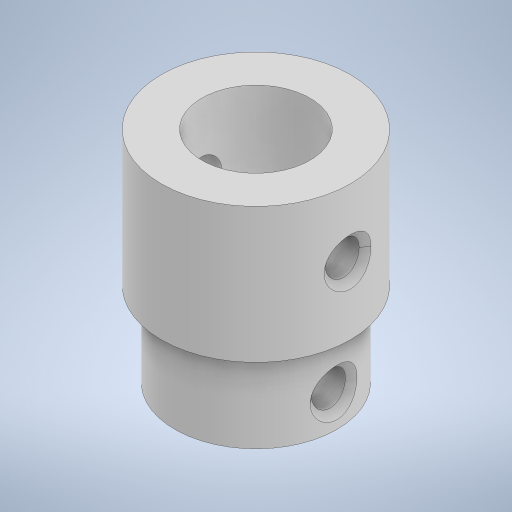
# Autodesk Inventor part: Acople2
Saved by Autodesk Inventor 2023 (Build 270158000, 158)
## iProperties
Created: 2022-12-24
Part Number: Acople2
Material: Genérico
Document SubType Name: Modeling
Designer: sergi
Density: 1 g/cm^3
Appearance: Valor por defecto
Author: sergi
Autodesk Inventor part; units mm, degrees
ref_plane "YZ Plane" through (0, 0, 0) normal (1, 0, 0) x (0, 1, 0)
ref_plane "XZ Plane" through (0, 0, 0) normal (0, 1, 0) x (-1, 0, 0)
ref_plane "XY Plane" through (0, 0, 0) normal (0, 0, 1) x (1, 0, 0)
sketch "Boceto1" plane through (0, 0, 0) normal (0, 1, 0) x (-1, 0, 0)
  circle A0 centre (0, 0) radius 7
  circle A1 centre (0, 0) radius 4
  dimension "d0" = 14
  dimension "d1" = 8
  constraints: 2 centre point, 2 coincident
  measures "d0" diameter of A0
  measures "d1" diameter of A1
extrude "Extrusión1" add sketch "Boceto1" along normal blind 10 contours A0 | A1
sketch "Boceto4" plane through (0, 10, 0) normal (0, 1, 0) x (1, 0, 0)
  circle A0 centre (0, 0) radius 4
  line L0 (0, 4) -> (0, -4)
  line L1 (-1.5, 4) -> (-1.5, -4)
  point P0 (-1.5, 3.7081)
  point P1 (-1.5, -3.7081)
  dimension "d21" = 8
  dimension "d45" = 1.5
  constraints: 4 end point, 2 point on circle, 1 centre point, 1 coincident, 1 parallel, 1 vertical
  measures "d21" diameter of A0
  measures "d45" distance between parallel lines of L0 L1
extrude "Extrusión2" cut sketch "Boceto4" against normal blind 8
sketch "Boceto5" plane through (0, 0, 0) normal (0, -1, 0) x (1, 0, 0)
  circle A0 centre (0, 0) radius 6
  dimension "d24" = 12
  constraints: 1 centre point, 1 coincident
  measures "d24" diameter of A0
extrude "Extrusión3" add sketch "Boceto5" along normal blind 6.25
sketch "Boceto11" plane through (0, 0, 0) normal (1, 0, 0) x (0, 1, 0)
  line L0 (-1.5, 0) -> (-1.5, 2.5882)
  line L1 (-1.5, 0) -> (-1.5, 2.5882)
  line L2 (0, 0) -> (-1.5, 0)
  line L3 (-4.85, 0) -> (-4.85, 0) projected
  line L4 (-1.5, -4) -> (-1.5, 4)
  line L5 (-6.25, 6) -> (-6.25, -6) projected
  line L6 (-1.5, 0) -> (-6.25, 0)
  circle A0 centre (-3.875, 0) radius 1.25
  dimension "d59" = 2.5
  constraints: 10 end point, 3 vertical, 2 midpoint, 1 centre point, 1 horizontal, 4 other
  measures "d59" diameter of A0
extrude "Extrusión9" cut sketch "Boceto11" along normal through all
sketch "Boceto12" plane through (0, -6.25, 0) normal (0, -1, 0) x (1, 0, 0)
  circle A0 centre (0, 0) radius 6 projected
  constraints: 1 coincident
hole "Agujero3" at (0, -6.25, 0) direction (0, 1, 0) diameter 3.5 depth 8 tip angle 118
sketch "Boceto14" plane through (0, 0, 0) normal (1, 0, 0) x (0, 1, 0)
  line L0 (10, -7) -> (10, 7) projected
  line L1 (10, 0) -> (0, 0)
  circle A0 centre (5, 0) radius 1.25
  dimension "d75" = 2.5
  constraints: 2 end point, 2 midpoint, 1 centre point, 1 horizontal
  measures "d75" diameter of A0
hole "Agujero5" at (0, 5, 0) direction (-1, 0, 0) diameter 2.5 end through all both
chamfer "Chaflán1" distance 1 angle 45 1 edges at (0, -6.25, 1.75)
chamfer "Chaflán2" distance 0.5 angle 45 3 edges at (6.8875, 4.9978, 1.25) (5.8683, -3.8751, -1.25) (5.8683, -3.875, 1.25)
